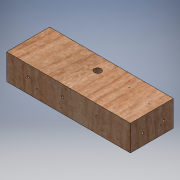
# Autodesk Inventor part: licht_150_support_right
Saved by Autodesk Inventor 2016 SP2 (Build 200236200, 236)
## iProperties
Created: 2018-01-11
Part Number: licht_150_support_right
Material: Spanplatte
Document SubType Name: Modeling
Designer: schueler
Density: 1 g/cm^3
Appearance: Birke - natur- poliert
Mass: 213.378 g
Surface Area: 284.671 cm^2
Volume: 213.378 cm^3
Author: schueler
Autodesk Inventor part; units mm, degrees
ref_plane "YZ Plane" through (0, 0, 0) normal (1, 0, 0) x (0, 1, 0)
ref_plane "XZ Plane" through (0, 0, 0) normal (0, 1, 0) x (-1, 0, 0)
ref_plane "XY Plane" through (0, 0, 0) normal (0, 0, 1) x (1, 0, 0)
sketch "Skizze1" plane through (0, 0, 0) normal (0, 0, 1) x (1, 0, 0)
  line L0 (0, 0) -> (144, 0)
  line L1 (144, 50) -> (0, 50)
  line L2 (72, 50) -> (72, 0) construction
  circle A0 centre (72, 34) radius 4
  line L3 (0, 50) -> (0, 0)
  line L4 (144, 0) -> (144, 50)
  line L5 (0, 20) -> (144, 20) construction
  line L6 (0, 34) -> (144, 34) construction
  circle A1 centre (105, 20) radius 1.5
  circle A2 centre (25, 20) radius 1.5
  circle A3 centre (65, 20) radius 1.5
  dimension "d17" = 8
  dimension "d207" = 50
  dimension "d224" = 144
  dimension "d225" = 20
  dimension "d226" = 34
  dimension "d228" = 3
  dimension "d229" = 3
  dimension "d232" = 3
  dimension "d233" = 7
  dimension "d234" = 40
  dimension "d235" = 40
  constraints: 14 end point, 8 point on line, 4 centre point, 3 midpoint, 2 horizontal, 2 parallel, 2 perpendicular, 1 vertical
  measures "d17" diameter of A0
  measures "d207" distance of L1.end L0.start
  measures "d224" distance between parallel lines of L4 L3
  measures "d225" distance between parallel lines of L5 L0
  measures "d226" distance between parallel lines of L6 L0
  measures "d228" diameter of A1
  measures "d229" diameter of A2
  measures "d232" diameter of A3
  measures "d233" distance from line of L2 A3.centre
  measures "d234" distance of A2.centre A3.centre
  measures "d235" distance of A1.centre A3.centre
extrude "Extrusion1" add sketch "Skizze1" along normal blind 30 contours L3 L1 L4 L0 | A1 | A2 | A3
sketch "Skizze7" plane through (0, 0, 0) normal (0, 0, -1) x (-1, 0, 0)
  line L0 (0, 0) -> (-144, 0) construction
  line L1 (-144, 50) -> (0, 50) construction
  line L2 (-144, 0) -> (-144, 50) construction
  line L3 (0, 50) -> (0, 0) construction
  line L4 (-144, 0) -> (-144, 50) projected
  line L5 (-144, 20) -> (0, 20) construction
  line L6 (0, 0) -> (-144, 0) construction
  line L7 (-72, 0) -> (-72, 50) construction
  point P0 (-79, 20)
  point P1 (-119, 20)
  point P2 (-39, 20)
  dimension "d236" = 7
  dimension "d237" = 20
  dimension "d238" = 40
  dimension "d239" = 40
  constraints: 5 point on line, 4 end point, 2 midpoint, 1 perpendicular
  measures "d236" distance from line of L7 point (-79, 20)
  measures "d237" distance between parallel lines of L5 L0
  measures "d238" distance of point (-79, 20) point (-119, 20)
  measures "d239" distance of point (-79, 20) point (-39, 20)
hole "Bohrung19" at (79, 20, 0) at (119, 20, 0) at (39, 20, 0) direction (0, 0, 1) diameter 2.5 depth 25 tip angle 118
sketch "Skizze8" plane through (0, 0, 0) normal (0, -1, 0) x (1, 0, 0)
  line L0 (144, 0) -> (144, 30) construction
  line L1 (0, 30) -> (144, 30) construction
  line L2 (0, 0) -> (144, 0) construction
  line L3 (144, 0) -> (144, 30) construction
  line L4 (0, 30) -> (144, 30) construction
  line L5 (0, 0) -> (0, 30) construction
  line L6 (144, 17) -> (0, 17) construction
  line L7 (25, 30) -> (25, 0) construction
  line L8 (0, 0) -> (144, 0) construction
  point P0 (25, 17)
  point P1 (65, 17)
  point P2 (105, 17)
  dimension "d247" = 17
  dimension "d248" = 25
  dimension "d249" = 40
  dimension "d250" = 40
  constraints: 8 point on line, 4 end point, 2 perpendicular
  measures "d247" distance between parallel lines of L2 L6
  measures "d248" distance between parallel lines of L5 L7
  measures "d249" distance from line of L7 point (65, 17)
  measures "d250" distance of point (65, 17) point (105, 17)
hole "Bohrung20" at (25, 0, 17) at (65, 0, 17) at (105, 0, 17) direction (0, 1, 0) diameter 2.5 depth 30 tip angle 118
sketch "Skizze9" plane through (144, 0, 0) normal (1, 0, 0) x (0, 0, -1)
  line L0 (0, 0) -> (0, 50) construction
  line L1 (0, 50) -> (-30, 50) construction
  line L2 (-30, 0) -> (-30, 50) construction
  line L3 (0, 0) -> (-30, 0) construction
  line L4 (0, 0) -> (-30, 0) construction
  line L5 (-13, 0) -> (-13, 50) construction
  point P0 (-13, 14)
  point P1 (-13, 39)
  dimension "d258" = 13
  dimension "d259" = 14
  dimension "d261" = 25
  constraints: 4 point on line, 2 end point, 1 vertical
  measures "d258" distance between parallel lines of L0 L5
  measures "d259" distance from line of L3 point (-13, 14)
  measures "d261" distance of point (-13, 14) point (-13, 39)
hole "Bohrung21" at (144, 14, 13) at (144, 39, 13) direction (-1, 0, 0) diameter 2.5 depth 30 tip angle 118
